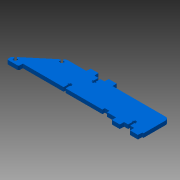
# Autodesk Inventor part: boardCaseSide
Saved by Autodesk Inventor 2013 (Build 170138000, 138)
## iProperties
Created: 2015-01-14
Part Number: boardCaseSide
Material: Generic
Document SubType Name: Modeling
Designer: dzban
Density: 1 g/cm^3
Author: dzban
Autodesk Inventor part; units mm, degrees
ref_plane "YZ Plane" through (0, 0, 0) normal (1, 0, 0) x (0, 1, 0)
ref_plane "XZ Plane" through (0, 0, 0) normal (0, 1, 0) x (-1, 0, 0)
ref_plane "XY Plane" through (0, 0, 0) normal (0, 0, 1) x (1, 0, 0)
sketch "Sketch1" plane through (0, 0, 0) normal (0, 0, 1) x (1, 0, 0)
  line L0 (-39.5101, 21.6819) -> (-39.5101, 14.6819)
  line L1 (-39.5101, 14.6819) -> (-38.2601, 14.6819)
  line L2 (-38.2601, 14.6819) -> (-38.2601, 12.8819)
  line L3 (-38.2601, 12.8819) -> (-39.5101, 12.8819)
  line L4 (-39.5101, 12.8819) -> (-39.5101, 11.0819)
  line L5 (-39.5101, 11.0819) -> (-42.5101, 11.0819)
  line L6 (-42.5101, 11.0819) -> (-42.5101, 12.8819)
  line L7 (-42.5101, 12.8819) -> (-43.7601, 12.8819)
  line L8 (-43.7601, 12.8819) -> (-43.7601, 14.6819)
  line L9 (-43.7601, 14.6819) -> (-42.5101, 14.6819)
  line L10 (-42.5101, 14.6819) -> (-42.5101, 21.6819)
  line L11 (-42.5101, 21.6819) -> (-48.6101, 21.6819)
  line L12 (-48.6101, 21.6819) -> (-48.9101, 28.0819)
  line L13 (-48.9101, 28.0819) -> (-60.7101, 28.0819)
  line L14 (-60.7101, 28.0819) -> (-61.0101, 21.6819)
  line L15 (-61.0101, 21.6819) -> (-90.8101, 21.6819)
  line L16 (-90.8101, 21.6819) -> (-93.4912, 19.4321)
  line L17 (-93.4912, 19.4321) -> (-91.3057, 16.8276)
  line L18 (-91.3057, 16.8276) -> (-90.3482, 17.6311)
  line L19 (-90.3482, 17.6311) -> (-89.1912, 16.2522)
  line L20 (-89.1912, 16.2522) -> (-90.1487, 15.4487)
  line L21 (-90.1487, 15.4487) -> (-88.9917, 14.0698)
  line L22 (-88.9917, 14.0698) -> (-91.2898, 12.1415)
  line L23 (-91.2898, 12.1415) -> (-92.4469, 13.5203)
  line L24 (-92.4469, 13.5203) -> (-93.4044, 12.7169)
  line L25 (-93.4044, 12.7169) -> (-94.5614, 14.0957)
  line L26 (-94.5614, 14.0957) -> (-93.6039, 14.8992)
  line L27 (-93.6039, 14.8992) -> (-95.7894, 17.5038)
  line L28 (-95.7894, 17.5038) -> (-131.7932, -12.7071)
  line L29 (-131.7932, -12.7071) -> (-129.6078, -15.3116)
  line L30 (-129.6078, -15.3116) -> (-128.6502, -14.5082)
  line L31 (-128.6502, -14.5082) -> (-127.4932, -15.887)
  line L32 (-127.4932, -15.887) -> (-128.4508, -16.6905)
  line L33 (-128.4508, -16.6905) -> (-127.2937, -18.0694)
  line L34 (-127.2937, -18.0694) -> (-129.5919, -19.9978)
  line L35 (-129.5919, -19.9978) -> (-130.7489, -18.6189)
  line L36 (-130.7489, -18.6189) -> (-131.7064, -19.4224)
  line L37 (-131.7064, -19.4224) -> (-132.8635, -18.0435)
  line L38 (-132.8635, -18.0435) -> (-131.9059, -17.24)
  line L39 (-131.9059, -17.24) -> (-133.9788, -14.7696)
  line L40 (-133.9788, -14.7696) -> (-136.66, -17.0193)
  line L41 (-136.66, -17.0193) -> (-136.5205, -21.4818)
  arc A0 (-136.5205, -21.4818) -> (-134.5215, -23.4193) centre (-134.5215, -21.4193) ccw
  line L42 (-134.5215, -23.4193) -> (-120.7985, -23.4193)
  arc A1 (-120.7985, -23.4193) -> (-118.7994, -21.4818) centre (-120.7985, -21.4193) ccw
  line L43 (-118.7994, -21.4818) -> (-118.66, -17.0193)
  line L44 (-118.66, -17.0193) -> (-56.7602, -17.0193)
  line L45 (-56.7602, -17.0193) -> (-56.7602, -10.0193)
  line L46 (-56.7602, -10.0193) -> (-58.0102, -10.0193)
  line L47 (-58.0102, -10.0193) -> (-58.0102, -8.2193)
  line L48 (-58.0102, -8.2193) -> (-56.7602, -8.2193)
  line L49 (-56.7602, -8.2193) -> (-56.7602, -6.4193)
  line L50 (-56.7602, -6.4193) -> (-53.7602, -6.4193)
  line L51 (-53.7602, -6.4193) -> (-53.7602, -8.2193)
  line L52 (-53.7602, -8.2193) -> (-52.5102, -8.2193)
  line L53 (-52.5102, -8.2193) -> (-52.5102, -10.0193)
  line L54 (-52.5102, -10.0193) -> (-53.7602, -10.0193)
  line L55 (-53.7602, -10.0193) -> (-53.7602, -17.0193)
  line L56 (-53.7602, -17.0193) -> (2.24, -17.0193)
  line L57 (2.24, -17.0193) -> (2.24, -13.3193)
  line L58 (2.24, -13.3193) -> (9.24, -13.3193)
  line L59 (9.24, -13.3193) -> (9.24, -17.0193)
  line L60 (9.24, -17.0193) -> (22.885, -17.0193)
  line L61 (22.885, -17.0193) -> (23.185, -23.4193)
  line L62 (23.185, -23.4193) -> (34.985, -23.4193)
  line L63 (34.985, -23.4193) -> (35.285, -17.0193)
  line L64 (35.285, -17.0193) -> (41.385, -17.0193)
  line L65 (41.385, -17.0193) -> (41.385, -10.0193)
  line L66 (41.385, -10.0193) -> (40.135, -10.0193)
  line L67 (40.135, -10.0193) -> (40.135, -8.2193)
  line L68 (40.135, -8.2193) -> (41.385, -8.2193)
  line L69 (41.385, -8.2193) -> (41.385, -6.4193)
  line L70 (41.385, -6.4193) -> (44.385, -6.4193)
  line L71 (44.385, -6.4193) -> (44.385, -8.2193)
  line L72 (44.385, -8.2193) -> (45.635, -8.2193)
  line L73 (45.635, -8.2193) -> (45.635, -10.0193)
  line L74 (45.635, -10.0193) -> (44.385, -10.0193)
  line L75 (44.385, -10.0193) -> (44.385, -17.0193)
  line L76 (44.385, -17.0193) -> (50.485, -17.0193)
  line L77 (50.485, -17.0193) -> (50.785, -23.4193)
  line L78 (50.785, -23.4193) -> (62.585, -23.4193)
  line L79 (62.585, -23.4193) -> (62.885, -17.0193)
  line L80 (62.885, -17.0193) -> (64.695, -17.0193)
  line L81 (64.695, -17.0193) -> (64.695, -3.7245)
  line L82 (64.695, -3.7245) -> (64.695, -0.6157)
  line L83 (64.695, -0.6157) -> (64.695, 16.6819)
  arc A2 (64.695, 16.6819) -> (59.695, 21.6819) centre (59.695, 16.6819) ccw
  line L84 (59.695, 21.6819) -> (-21.0101, 21.6819)
  line L85 (-21.0101, 21.6819) -> (-21.3101, 28.0819)
  line L86 (-21.3101, 28.0819) -> (-33.1101, 28.0819)
  line L87 (-33.1101, 28.0819) -> (-33.4101, 21.6819)
  line L88 (-33.4101, 21.6819) -> (-39.5101, 21.6819)
  point P0 (0, 0)
  point P1 (0, 0)
  constraints: 178 end point, 6 point on circle, 3 centre point
extrude "Extrusion1" add sketch "Sketch1" along normal blind 6
body "Solid1"
